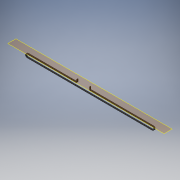
# Autodesk Inventor part: X-axis belt
Saved by Autodesk Inventor 2018 (Build 220112000, 112)
## iProperties
Created: 2017-11-20
Part Number: X-axis belt
Material: Rubber
Document SubType Name: Modeling
Designer: Gabriel Smolnycki
Density: 0.93 g/cm^3
Appearance: Rubber - Black
Author: Gabriel Smolnycki
Autodesk Inventor part; units mm, degrees
ref_plane "YZ Plane" through (0, 0, 0) normal (1, 0, 0) x (0, 1, 0)
ref_plane "XY Plane" through (0, 0, 0) normal (0, 0, 1) x (1, 0, 0)
sketch "Sketch1" plane through (0, 0, 0) normal (0, 0, 1) x (1, 0, 0)
  circle A0 centre (0, 0) radius 6.5 projected
  line L0 (-306, 8) -> (-306, 19) projected
  line L1 (-252, 19) -> (-252, 8) projected
  line L2 (-304, 8) -> (-304, 19) projected
  line L3 (-254, 8) -> (-254, 19) projected
  line L4 (-253, 19) -> (-253, 8)
  arc A1 (-253, 8) -> (-252, 7) centre (-252, 8) ccw
  line L5 (-252, 8) -> (-252, 7) construction
  line L6 (-252, 8) -> (-253, 8) construction
  arc A2 (0, -6.5) -> (0.0129, 6.5) centre (0, 0) ccw
  line L7 (-252, 7) -> (0.0129, 6.5)
  line L8 (0, -6.5) -> (-505, -5.3948)
  arc A3 (-498.6236, 1) -> (-498.7461, 2.244) centre (-505, 1) ccw projected
  arc A4 (-505, 7.3948) -> (-505, -5.3948) centre (-505, 1) ccw
  line L9 (-505, 7.3948) -> (-306, 7)
  line L10 (-305, 19) -> (-305, 8)
  arc A5 (-306, 7) -> (-305, 8) centre (-306, 8) ccw
  point P0 (0, 0)
  dimension "d0" = 2
  dimension "d1" = 1
  dimension "d3" = 90
  dimension "d6" = 2
  dimension "d15" = 1
  constraints: 14 end point, 10 point on circle, 4 centre point, 4 coincident, 2 tangent, 2 vertical, 1 concentric
  measures "d0" distance between parallel lines of L1 L3
  measures "d1" distance between parallel lines of L4 L3
  measures "d3" angle of L6 L5
  measures "d6" distance between parallel lines of L2 L0
  measures "d15" distance between parallel lines of L0 L10
ref_plane "Work Plane1" through (-253, 19, 0) normal (0, 1, 0) x (-1, 0, 0)
sketch "Sketch2" plane through (-253, 19, 0) normal (0, 1, 0) x (-1, 0, 0)
  line L0 (1, 11.1) -> (1, -4.9) projected
  line L1 (-1, -10.9) -> (-1, 10.1) projected
  line L2 (0.65, -2.4) -> (-0.65, -2.4)
  line L3 (-0.65, -2.4) -> (-0.65, 3.6)
  line L4 (-0.65, 3.6) -> (0.65, 3.6)
  line L5 (0.65, 3.6) -> (0.65, -2.4)
  point P0 (-253, 0)
  point P1 (0, -2.4)
  dimension "d9" = 2
  dimension "d10" = 1.3
  dimension "d11" = 1
  dimension "d12" = 6
  dimension "d13" = 2.4
  constraints: 8 end point, 2 parallel, 1 horizontal, 1 midpoint, 1 perpendicular
  measures "d9" distance between parallel lines of L1 L0
  measures "d10" distance of L3.end L4.end
  measures "d11" distance from line of point (0, -2.4) L0
  measures "d12" distance of L2.end L3.end
  measures "d13" distance from line of point (-253, 0) L2
sweep "Sweep1" add profiles "Sketch2" path "Sketch1" path curves L4 A1 L7 A2 L8 A4 L9 A5 L10
equation "\"d1\" = 0.5 * d0"
equation "\"d15\" = 0.5 * d6"
equation "\"d11\" = 0.5 * d9"
body "Solid1"
